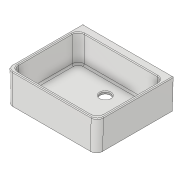
# Autodesk Inventor part: Sink 63220001
Saved by Autodesk Inventor 2018 (Build 220112000, 112)
## iProperties
Created: 2017-12-11
Part Number: Sink 63220001
Material: Concrete
Document SubType Name: Modeling
Designer: sawaiz
Density: 2.40731 g/cm^3
Appearance: Smooth - White
Author: sawaiz
Autodesk Inventor part; units mm, degrees
ref_plane "YZ Plane" through (0, 0, 0) normal (1, 0, 0) x (0, 1, 0)
ref_plane "XZ Plane" through (0, 0, 0) normal (0, 1, 0) x (-1, 0, 0)
ref_plane "XY Plane" through (0, 0, 0) normal (0, 0, 1) x (1, 0, 0)
sketch "Sketch1" plane through (0, 0, 0) normal (0, 1, 0) x (-1, 0, 0)
  line L0 (297.5, -250) -> (-297.5, -250)
  line L1 (-297.5, -250) -> (-297.5, 250)
  line L2 (-297.5, 250) -> (297.5, 250)
  line L3 (297.5, 250) -> (297.5, -250)
  line L4 (297.5, -250) -> (-297.5, 250) construction
  line L5 (-297.5, -250) -> (297.5, 250) construction
  point P0 (0, 0)
  point P1 (0, 0)
  dimension "d0" = 595
  dimension "d1" = 500
  constraints: 12 end point, 2 parallel, 1 coincident, 1 horizontal, 1 midpoint, 1 perpendicular
  measures "d0" distance of L0.start L0.end
  measures "d1" distance of L0.end L1.end
extrude "Extrusion1" add sketch "Sketch1" along normal blind 200
sketch "Sketch2" plane through (0, 200, 0) normal (0, 1, 0) x (1, 0, 0)
  line L0 (-277.5, -230) -> (277.5, -230)
  line L1 (277.5, -230) -> (277.5, 200)
  line L2 (277.5, 200) -> (-277.5, 200)
  line L3 (-277.5, 200) -> (-277.5, -230)
  line L4 (-277.5, -230) -> (-297.5, -230) construction
  line L5 (277.5, -230) -> (297.5, -230) construction
  line L6 (277.5, -230) -> (277.5, -250) construction
  line L7 (-297.5, -250) -> (297.5, -250) projected
  line L8 (297.5, -250) -> (297.5, 250) projected
  point P0 (0, 0)
  dimension "d4" = 555
  dimension "d5" = 430
  dimension "d12" = 20
  dimension "d13" = 595
  dimension "d14" = 20
  constraints: 14 end point, 3 horizontal, 2 equal length, 2 parallel, 1 perpendicular, 1 point on line, 1 vertical
  measures "d4" distance of L0.start L0.end
  measures "d5" distance between parallel lines of L0 L2
  measures "d12" distance between parallel lines of L1 L8
  measures "d13" distance of L7.start L7.end
  measures "d14" distance of L0.start L4.end
extrude "Extrusion2" cut sketch "Sketch2" against normal blind 180
sketch "Sketch3" plane through (-297.5, 0, 250) normal (0, 0, 1) x (1, 0, 0)
  line L0 (595, 0) -> (0, 0) projected
  line L1 (595, 0) -> (595, 200) projected
  line L2 (0, 200) -> (595, 200) projected
  line L3 (0, 0) -> (0, 200) projected
  line L4 (595, 200) -> (0, 200) projected
  line L5 (0, 200) -> (5, 0)
  line L6 (0, 0) -> (595, 0) projected
  line L7 (595, 200) -> (590, 0)
  line L8 (590, 0) -> (5, 0)
  line L9 (0, 200) -> (595, 200)
  point P0 (297.5, 0)
  dimension "d8" = 585
  constraints: 8 end point, 2 point on line, 1 collinear, 1 equal length, 1 perpendicular
  measures "d8" distance of L7.end L5.end
extrude "Extrusion3" cut sketch "Sketch3" against normal through all contours L0 L5 L2 L7 keep common part
fillet "Fillet1" radius 40 6 edges at (-277.5, 110, -200) (277.5, 110, -200) (295, 100, 250) (277.5, 110, 230) (-295, 100, 250) (-277.5, 110, 230)
fillet "Fillet2" radius 5 22 edges at (-265.7843, 200, -188.2843) (0, 200, -200) (265.7843, 200, -188.2843) (277.5, 200, 15) (265.7843, 200, 218.2843) (0, 200, 230) (-265.7843, 200, 218.2843) (-277.5, 200, 15) (-285.7806, 200, 238.2843) (0, 200, 250) (285.7806, 200, 238.2843) (297.5, 200, -20) (-297.5, 200, -20) (0, 200, -250) (295, 100, -250) (-295, 100, -250) (-280.7806, 0, 238.2843) (-292.5, 0, -20) (280.7806, 0, 238.2843) (292.5, 0, -20) (0, 0, 250) (0, 0, -250)
fillet "Fillet3" radius 10 8 edges at (-277.5, 20, 15) (-265.7843, 20, 218.2843) (0, 20, 230) (265.7843, 20, 218.2843) (277.5, 20, 15) (265.7843, 20, -188.2843) (0, 20, -200) (-265.7843, 20, -188.2843)
sketch "Sketch4" plane through (0, 20, 0) normal (0, 1, 0) x (1, 0, 0)
  line L0 (-297.3719, 245) -> (-297.3719, -210) projected
  line L1 (292.3734, 250) -> (-292.3734, 250) projected
  line L2 (297.3719, -210) -> (297.3719, 245) projected
  line L3 (267.5, 160) -> (267.5, -190) projected
  line L4 (-267.5, -190) -> (-267.5, 160) projected
  point P0 (0, 0)
  point P1 (0, 100)
  dimension "d18" = 150
  dimension "d27" = 535
  dimension "d28" = 267.5
  measures "d18" distance from line of L1 point (0, 100)
  measures "d27" distance between parallel lines of L3 L4
  measures "d28" distance from line of L3 point (0, 100)
hole "Hole1" at (0, 20, -100) direction (0, -1, 0) diameter 65 end through all
fillet "Fillet4" radius 5 2 edges at (0, 20, -132.5) (0, 0, -132.5)
equation "\"d12\" = -0.5 * d4 + 0.5 * d13"
equation "\"d14\" = d12"
equation "\"d28\" = 0.5 * d27"
body "Solid1"
